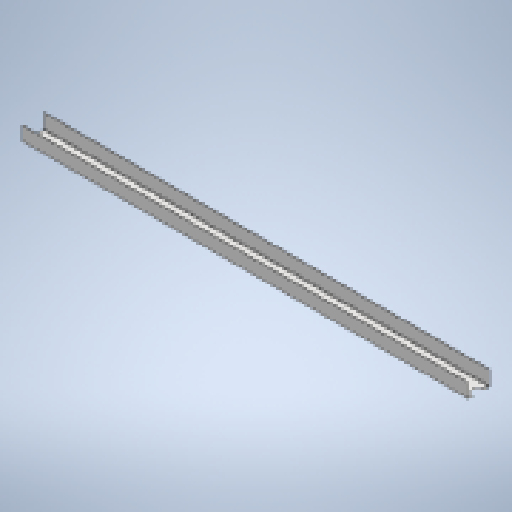
# Autodesk Inventor part: MSC 081 pillar 1
Saved by Autodesk Inventor 2025 (Build 290162010, 162A)
## iProperties
Created: 2024-06-25
Part Number: MSC 081 pillar 1
Material: Stainless Steel
Document SubType Name: Sheet Metal
Designer: admin
Density: 8 g/cm^3
Sheet Metal Rule: AISI304 3mm Die 32
Appearance: Default
Author: admin
Autodesk Inventor part; units mm, degrees
ref_plane "YZ Plane" through (0, 0, 0) normal (1, 0, 0) x (0, 1, 0)
ref_plane "XZ Plane" through (0, 0, 0) normal (0, 1, 0) x (-1, 0, 0)
ref_plane "XY Plane" through (0, 0, 0) normal (0, 0, 1) x (1, 0, 0)
sketch3d "3D Sketch1"
sketch "Sketch1" plane through (0, 0, 0) normal (0, 0, 1) x (1, 0, 0)
  line L0 (-1500, 75) -> (1500, 75)
  line L1 (1500, 75) -> (1500, -75)
  line L2 (1500, -75) -> (-1500, -75)
  line L3 (-1500, -75) -> (-1500, 75)
  line L4 (-1500, 75) -> (1500, -75) construction
  line L5 (1500, 75) -> (-1500, -75) construction
  point P0 (0, 0)
  dimension "d5" = 3000
  dimension "d30" = 150
  measures "d5" distance of L1.end L2.end
  measures "d30" distance of L2.end L0.start
extrude "Plate1" add sketch "Sketch1" along normal blind 3
sketch "Sketch6" plane through (1500, -72, 0) normal (0, -1, 0) x (1, 0, 0)
  line L0 (-3000, 0) -> (0, 0)
  line L1 (0, 0) -> (0, 80)
  line L2 (0, 80) -> (-3000, 80)
  line L3 (-3000, 80) -> (-3000, 0)
  constraints: 6 end point, 1 horizontal, 1 perpendicular, 1 vertical
edge flange "Flange4" height 80 angle 90 thickness 3 bend radius 5 thickness toward (0, -1, 0) relief round relief width 3 relief depth 1.5 corner gap 5 corner form 0 edges at (0, -75, 3) (0, 75, 3) wall of the first edge with corners at (-1500, -72, 0) (1500, -72, 0) (1500, -72, 80) (-1500, -72, 80)
bend "Bend4"
corner "Corner4"
sketch "Sketch7" plane through (0, 0, 3) normal (0, 0, 1) x (1, 0, 0)
  circle A0 centre (1500, 0) radius 40
  line L0 (1500, 67) -> (1500, -67) projected
  point P0 (0, 0)
  point P1 (1500, -40)
  point P2 (1500, 40)
  dimension "d70" = 80
  constraints: 1 centre point, 1 midpoint
  measures "d70" diameter of A0
extrude "Extrusion2" cut sketch "Sketch7" against normal through all contours L0 A0 picked at (1480.2577, -5.8053)
equation "\"d6\" = Thickness"
equation "\"d60\" = BendReliefWidth"
equation "\"d61\" = BendReliefDepth"
equation "\"d62\" = MinimumRemnant"
equation "\"d63\" = TransitionRadius"
equation "\"d66\" = BendRadius"
equation "\"d67\" = CornerReliefSize"
equation "\"d68\" = GapSize"
equation "\"d69\" = JacobiRadiusSize"
equation "\"BendReliefWidth\" = Thickness"
equation "\"BendReliefDepth\" = 0.5 * Thickness"
equation "\"CornerReliefSize\" = 4 * Thickness"
equation "\"MinimumRemnant\" = 2 * Thickness"
equation "\"TransitionRadius\" = BendRadius"
equation "\"JacobiRadiusSize\" = BendRadius"
equation "\"GapSize\" = Thickness"
equation "\"Thickness\" = 3"
equation "\"BendRadius\" = 5"
body "Solid1"
